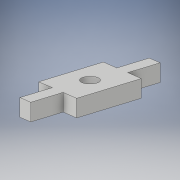
# Autodesk Inventor part: 小零件1
Saved by Autodesk Inventor 2017 (Build 210142000, 142)
## iProperties
Part Number: 小零件1
Material: 一般
Document SubType Name: Modeling
Designer: User
Density: 1 g/cm^3
Appearance: 預設
Author: User
Autodesk Inventor part; units mm, degrees
ref_plane "YZ Plane" through (0, 0, 0) normal (1, 0, 0) x (0, 1, 0)
ref_plane "XZ Plane" through (0, 0, 0) normal (0, 1, 0) x (-1, 0, 0)
ref_plane "XY Plane" through (0, 0, 0) normal (0, 0, 1) x (1, 0, 0)
sketch "草圖1" plane through (0, 0, 0) normal (0, 1, 0) x (-1, 0, 0)
  line L0 (4.2, 0) -> (4.2, -6)
  line L1 (4.2, -6) -> (0, -6)
  line L2 (0, -6) -> (1.2, -6)
  line L3 (1.2, -6) -> (1.2, -12)
  line L4 (1.2, -12) -> (0, -12)
  line L5 (-4.2, 0) -> (-4.2, -6)
  line L6 (-4.2, -6) -> (0, -6)
  line L7 (0, -6) -> (-1.2, -6)
  line L8 (-1.2, -6) -> (-1.2, -12)
  line L9 (-1.2, -12) -> (0, -12)
  line L10 (4.2, 0) -> (4.2, 6)
  line L11 (4.2, 6) -> (0, 6)
  line L12 (0, 6) -> (1.2, 6)
  line L13 (1.2, 6) -> (1.2, 12)
  line L14 (1.2, 12) -> (0, 12)
  line L15 (-4.2, 0) -> (-4.2, 6)
  line L16 (-4.2, 6) -> (0, 6)
  line L17 (0, 6) -> (-1.2, 6)
  line L18 (-1.2, 6) -> (-1.2, 12)
  line L19 (-1.2, 12) -> (0, 12)
  circle A0 centre (0, 0) radius 1.5
  dimension "d0" = 6
  dimension "d1" = 1.2
  dimension "d2" = 3
  dimension "d3" = 6
  dimension "d4" = 3
  constraints: 40 end point, 1 centre point, 1 coincident, 1 horizontal, 1 parallel, 1 perpendicular
  measures "d0" distance of L0.start L0.end
  measures "d1" distance of L3.end L4.end
  measures "d2" distance between parallel lines of L3 L0
  measures "d3" distance of L2.end L3.end
  measures "d4" diameter of A0
extrude "擠出1" add sketch "草圖1" along normal mid plane 3
